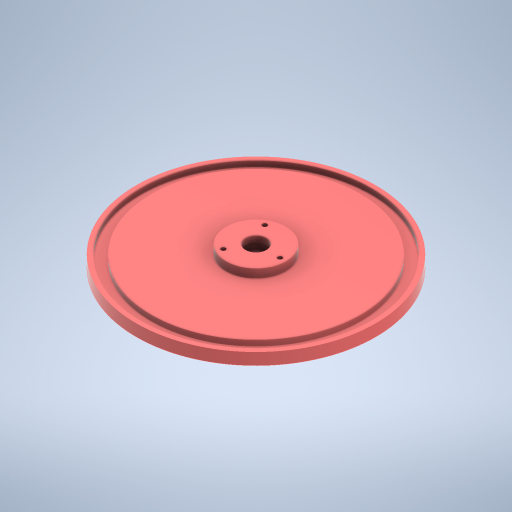
# Autodesk Inventor part: 007
Saved by Autodesk Inventor 2023 (Build 270158000, 158)
## iProperties
Created: 2021-11-05
Part Number: 007
Material: Stainless Steel, 440C
Document SubType Name: Modeling
Designer: vinicius.miguel
Density: 7.75 g/cm^3
Appearance: Smooth - Red
Mass: 141.616 g
Surface Area: 120.59 cm^2
Volume: 18.2731 cm^3
Author: vinicius.miguel
Autodesk Inventor part; units mm, degrees
ref_plane "YZ Plane" through (0, 0, 0) normal (1, 0, 0) x (0, 1, 0)
ref_plane "XZ Plane" through (0, 0, 0) normal (0, 1, 0) x (-1, 0, 0)
ref_plane "XY Plane" through (0, 0, 0) normal (0, 0, 1) x (1, 0, 0)
sketch "Sketch1" plane through (0, 0, 0) normal (0, 0, 1) x (1, 0, 0)
  line L0 (0, 0) -> (0, 5) construction
  line L1 (-40, 4) -> (-40, 0)
  line L2 (-40, 0) -> (-3.5, 0)
  line L3 (-38.5, 4) -> (-38.5, 2)
  line L4 (-38.5, 2) -> (-35, 2)
  line L5 (-35, 2) -> (-35, 4)
  line L6 (-10, 4) -> (-35, 4)
  line L7 (-38.5, 4) -> (-40, 4)
  line L8 (-3.5, 5) -> (-4.5, 5)
  line L9 (-4.5, 5) -> (-4.5, 2)
  line L10 (-4.5, 2) -> (-3.5, 2)
  line L11 (-3, 2.9949) -> (3, 2.9949)
  line L12 (3, 2.9949) -> (3, 2.0051)
  line L13 (3, 2.0051) -> (-3, 2.0051)
  line L14 (-3, 2.0051) -> (-3, 2.9949)
  line L15 (-3, 2.9949) -> (3, 2.0051) construction
  line L16 (3, 2.9949) -> (-3, 2.0051) construction
  line L17 (-10, 4) -> (-10, 7)
  line L18 (-10, 7) -> (-3.5, 7)
  line L19 (-3.5, 7) -> (-3.5, 5)
  line L20 (-3.5, 0) -> (-3.5, 2)
  point P0 (0, 2.5)
  dimension "d0" = 4
  dimension "d3" = 80
  dimension "d6" = 3.5
  dimension "d7" = 2
  dimension "d15" = 70
  dimension "d16" = 6
  dimension "d17" = 1.5
  dimension "d18" = 3
  dimension "d33" = 3
  dimension "d34" = 20
  dimension "d35" = 7
  constraints: 42 end point, 13 perpendicular, 4 vertical, 3 horizontal alignment, 3 midpoint, 2 horizontal, 2 parallel, 1 collinear, 1 vertical alignment
  measures "d0" distance of L1.start L1.end
  measures "d3" diameter of L1 L0
  measures "d6" distance of L3.end L4.end
  measures "d7" distance of L4.end L5.end
  measures "d15" diameter of L5 L0
  measures "d16" distance of L12.end L13.end
  measures "d17" distance between parallel lines of L9 L14
  measures "d18" distance of L8.end L9.end
  measures "d33" distance of L6.start L17.end
  measures "d34" diameter of L17 L0
  measures "d35" diameter of L19 L0
revolve "Revolution1" add sketch "Sketch1" angle 360 about axis through (0, 0, 0) along (0, 1, 0) contours L7 L3 L4 L5 L6 L17 L18 L19 L8 L9 L10 L20 L2 L1
sketch "Sketch3" plane through (0, 7, 0) normal (0, 1, 0) x (1, 0, 0)
  circle A0 centre (0, 0) radius 3.5 projected
  point P0 (8, 0)
  dimension "d36" = 8
  constraints: 1 horizontal alignment
  measures "d36" distance of A0.centre point (8, 0)
hole "Hole1" at (8, 7, 0) direction (0, -1, 0) diameter 1.567 depth 5 tip angle 118 thread size "M2x0.4" class "6H" standard "ISO Metric profile"
pattern_circular "Circular Pattern2" count 3 over 360 about axis through (0, 5.5, 0) along (0, 1, 0) of "Hole1"
body "Solid1"
